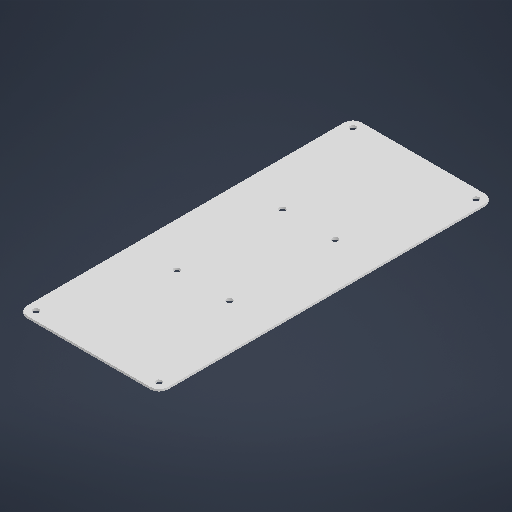
# Autodesk Inventor part: brainmount(pocketlater)
Saved by Autodesk Inventor 2025.2 (Build 292293000, 293)
## iProperties
Created: 2025-03-30
Part Number: brainmount(pocketlater)
Material: Generic
Document SubType Name: Modeling
Designer: Jahan
Density: 1 g/cm^3
Appearance: Default
Author: Jahan
Autodesk Inventor part; units mm, degrees
ref_plane "YZ Plane" through (0, 0, 0) normal (1, 0, 0) x (0, 1, 0)
ref_plane "XZ Plane" through (0, 0, 0) normal (0, 1, 0) x (-1, 0, 0)
ref_plane "XY Plane" through (0, 0, 0) normal (0, 0, 1) x (1, 0, 0)
sketch "Sketch1" plane through (0, 0, 0) normal (0, 1, 0) x (-1, 0, 0)
  circle A0 centre (0, 0) radius 2.1844
  circle A1 centre (0, -228.6) radius 2.1844
  circle A2 centre (88.9, 0) radius 2.1844
  circle A3 centre (88.9, -228.6) radius 2.1844
  circle A4 centre (63.5, -76.2) radius 2.1844
  circle A5 centre (63.5, -152.4) radius 2.1844
  circle A6 centre (25.4, -152.4) radius 2.1844
  circle A7 centre (25.4, -76.2) radius 2.1844
  line L0 (95.25, 0) -> (95.25, -228.6)
  line L1 (88.9, -234.95) -> (0, -234.95)
  line L2 (-6.35, -228.6) -> (-6.35, 0)
  line L3 (0, 6.35) -> (88.9, 6.35)
  arc A8 (95.25, 0) -> (88.9, 6.35) centre (88.9, 0) ccw
  arc A9 (88.9, -234.95) -> (95.25, -228.6) centre (88.9, -228.6) ccw
  arc A10 (-6.35, -228.6) -> (0, -234.95) centre (0, -228.6) ccw
  arc A11 (0, 6.35) -> (-6.35, 0) centre (0, 0) ccw
  line L4 (88.9, 0) -> (88.9, -228.6)
  line L5 (0, 0) -> (0, -228.6)
  point P0 (44.45, -114.3)
  point P1 (44.45, -114.3)
  dimension "d0" = 4.3688
  dimension "d2" = 4.3688
  dimension "d7" = 4.3688
  dimension "d8" = 4.3688
  dimension "d15" = 4.3688
  dimension "d16" = 4.3688
  dimension "d17" = 4.3688
  dimension "d18" = 4.3688
  constraints: 12 centre point, 12 end point, 8 point on circle, 5 coincident, 1 perpendicular, 1 vertical, 7 other
  measures "d0" diameter of A0
  measures "d2" diameter of A1
  measures "d7" diameter of A2
  measures "d8" diameter of A3
  measures "d15" diameter of A4
  measures "d16" diameter of A5
  measures "d17" diameter of A6
  measures "d18" diameter of A7
extrude "Extrusion1" add sketch "Sketch1" along normal blind 1.5875
body "Solid1"
